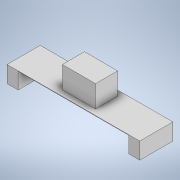
# Autodesk Inventor part: bridgeTest
Saved by Autodesk Inventor 2020 (Build 240168000, 168)
## iProperties
Created: 2021-04-27
Part Number: bridgeTest
Material: Generic
Document SubType Name: Modeling
Designer: dkiiv
Density: 1 g/cm^3
Appearance: Default
Author: dkiiv
Autodesk Inventor part; units mm, degrees
ref_plane "YZ Plane" through (0, 0, 0) normal (1, 0, 0) x (0, 1, 0)
ref_plane "XZ Plane" through (0, 0, 0) normal (0, 1, 0) x (-1, 0, 0)
ref_plane "XY Plane" through (0, 0, 0) normal (0, 0, 1) x (1, 0, 0)
sketch "Sketch1" plane through (0, 0, 0) normal (0, 0, 1) x (1, 0, 0)
  line L0 (0, 0) -> (5, 0)
  line L1 (5, 0) -> (5, 7.3)
  line L2 (5, 7.5) -> (0, 7.5)
  line L3 (0, 7.5) -> (0, 0)
  line L4 (5, 7.5) -> (55, 7.5)
  line L5 (55, 7.5) -> (55, 7.3)
  line L6 (55, 7.3) -> (5, 7.3)
  line L7 (5, 7.3) -> (5, 7.5)
  line L8 (55, 7.5) -> (60, 7.5)
  line L9 (60, 7.5) -> (60, 0)
  line L10 (60, 0) -> (55, 0)
  line L11 (55, 0) -> (55, 7.5)
  dimension "d0" = 5
  dimension "d1" = 7.5
  dimension "d2" = 50
  dimension "d3" = 0.2
  dimension "d4" = 5
  dimension "d5" = 7.5
  constraints: 24 end point, 6 parallel, 3 horizontal, 3 perpendicular
  measures "d0" distance of L2.end L2.start
  measures "d1" distance of L2.start L0.end
  measures "d2" distance of L1.end L5.end
  measures "d3" distance of L4.end L5.end
  measures "d4" distance of L9.end L10.end
  measures "d5" distance of L8.end L9.end
extrude "Extrusion1" add sketch "Sketch1" along normal blind 15
sketch "Sketch2" plane through (0, 7.5, 0) normal (0, 1, 0) x (1, 0, 0)
  line L0 (0, 0) -> (0, -15) projected
  line L1 (0, -7.5) -> (30, -7.5) construction
  line L2 (60, 0) -> (60, -15) projected
  line L3 (30, -7.5) -> (30, 0) construction
  line L4 (5, 0) -> (55, 0) projected
  line L5 (22.5, -12.5) -> (37.5, -12.5)
  line L6 (37.5, -12.5) -> (37.5, -2.5)
  line L7 (37.5, -2.5) -> (22.5, -2.5)
  line L8 (22.5, -2.5) -> (22.5, -12.5)
  line L9 (22.5, -12.5) -> (37.5, -2.5) construction
  line L10 (37.5, -12.5) -> (22.5, -2.5) construction
  dimension "d8" = 30
  dimension "d9" = 15
  dimension "d10" = 10
  constraints: 16 end point, 4 midpoint, 2 parallel, 2 perpendicular, 1 horizontal
  measures "d8" distance of L1.start L1.end
  measures "d9" distance of L7.end L6.end
  measures "d10" distance of L6.end L5.end
extrude "Extrusion2" add sketch "Sketch2" along normal blind 10
body "Solid1"
